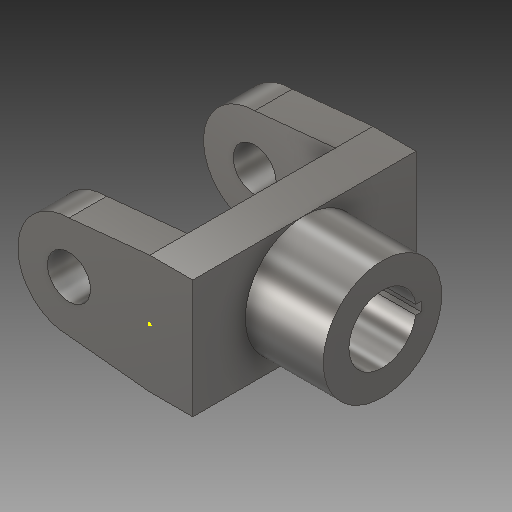
# Autodesk Inventor part: Fork 2 Off
Saved by Autodesk Inventor 2018 (Build 220112000, 112)
## iProperties
Created: 2018-09-13
Part Number: Fork 2 Off
Material: Stainless Steel
Document SubType Name: Modeling
Designer: Ajay Sharma
Density: 8 g/cm^3
Appearance: Semi-Polished
Author: Ajay Sharma
Autodesk Inventor part; units mm, degrees
ref_plane "YZ Plane" through (0, 0, 0) normal (1, 0, 0) x (0, 1, 0)
ref_plane "XZ Plane" through (0, 0, 0) normal (0, 1, 0) x (-1, 0, 0)
ref_plane "XY Plane" through (0, 0, 0) normal (0, 0, 1) x (1, 0, 0)
sketch "Sketch1" plane through (0, 0, 0) normal (1, 0, 0) x (0, 1, 0)
  line L0 (0, 116.2) -> (0, -116.2) projected
  line L1 (-61.6, 0) -> (61.6, 0) projected
  line L2 (44, 83) -> (-44, 83)
  line L3 (-44, 83) -> (-44, -83)
  line L4 (-44, -83) -> (44, -83)
  line L5 (44, -83) -> (44, 83)
  point P0 (0, 0)
  dimension "d0" = 166
  dimension "d1" = 88
  constraints: 8 end point, 2 parallel, 1 horizontal, 1 perpendicular, 2 other
  measures "d0" distance of L4.end L2.start
  measures "d1" distance of L2.start L2.end
extrude "Extrusion1" add sketch "Sketch1" along normal blind 32
sketch "Sketch2" plane through (32, 0, 0) normal (1, 0, 0) x (0, 0, -1)
  line L0 (-116.2, 0) -> (116.2, 0) projected
  line L1 (0, -61.6) -> (0, 61.6) projected
  circle A0 centre (0, 0) radius 44
  arc A1 (24.7538, 3.5) -> (24.7538, -3.5) centre (0, 0) ccw
  line L2 (25, 0) -> (29, 0)
  line L3 (29, 0) -> (29, 3.5)
  line L4 (29, 3.5) -> (24.7538, 3.5)
  arc A2 (24.7538, 3.5) -> (24.7538, -3.5) centre (0, 0) ccw
  line L5 (29, 0) -> (29, -3.5)
  line L6 (29, -3.5) -> (24.7538, -3.5)
  dimension "d4" = 88
  dimension "d5" = 50
  dimension "d6" = 4
  dimension "d7" = 3.5
  constraints: 10 end point, 4 point on circle, 3 centre point, 2 coincident, 2 perpendicular, 2 point on line, 2 symmetric about line, 1 other
  measures "d4" diameter of A0
  measures "d5" diameter of A1
  measures "d6" distance of L2.start L2.end
  measures "d7" distance of L2.end L3.end
extrude "Extrusion2" add sketch "Sketch2" along normal blind 58 contours L3 L4 A1 L1 A0 L0 | L0 A0 L1 A1 L6 L5 | A1 L1 A0 L0 | L0 A0 L1 A1
sketch "Sketch3" plane through (0, 0, 0) normal (-1, 0, 0) x (0, 0, 1)
  line L0 (-116.2, 0) -> (116.2, 0) projected
  line L1 (0, 61.6) -> (0, -61.6) projected
  line L2 (-83, 44) -> (83, 44) projected
  line L3 (83, -44) -> (-83, -44) projected
  line L4 (-83, 44) -> (-55, 44)
  line L5 (-55, 44) -> (-55, -44)
  line L6 (-55, -44) -> (-83, -44)
  line L7 (-83, -44) -> (-83, 44)
  line L8 (0, 44) -> (83, 44) projected
  line L9 (83, 44) -> (55, 44)
  line L10 (55, 44) -> (55, -44)
  line L11 (55, -44) -> (83, -44)
  line L12 (83, -44) -> (83, 44)
  point P0 (0, 0)
  dimension "d10" = 28
  dimension "d11" = 28
  constraints: 16 end point, 4 parallel, 2 horizontal, 2 perpendicular, 2 point on line
  measures "d10" distance from line of L5 L2.start
  measures "d11" distance from line of L10 L2.end
extrude "Extrusion3" add sketch "Sketch3" along normal blind 98 contours L7 L2 L5 L0 | L0 L5 L3 L7 | L10 L2 L12 L0 | L0 L12 L3 L10
sketch "Sketch4" plane through (32, -44, 83) normal (0, 0, 1) x (1, 0, 0)
  point P0 (-32, 44)
sketch "Sketch5" plane through (32, -44, 83) normal (0, 0, 1) x (1, 0, 0)
  circle A0 centre (-92, 44) radius 38
  line L0 (-92, 6) -> (-32, 0)
  line L1 (-130, 0) -> (0, 0) projected
  line L2 (-32, 88) -> (-32, 0) projected
  line L3 (-32, 88) -> (-92, 82)
  line L4 (0, 88) -> (-130, 88) projected
  line L5 (-32, 88) -> (-130, 88)
  line L6 (-130, 0) -> (-130, 88) projected
  line L7 (-130, 88) -> (-130, 0)
  line L8 (-130, 0) -> (-32, 0)
  point P0 (-32, 44)
  dimension "d14" = 76
  constraints: 10 end point, 2 collinear, 2 point on circle, 1 centre point, 1 perpendicular, 1 point on line
  measures "d14" diameter of A0
extrude "Extrusion4" cut sketch "Sketch5" against normal through all contours A0 L6 L4 L3 | L0 L1 L6 A0
sketch "Sketch6" plane through (32, -44, 83) normal (0, 0, 1) x (1, 0, 0)
  arc A0 (-92, 82) -> (-92, 6) centre (-92, 44) ccw projected
  circle A1 centre (-92, 44) radius 16
  point P0 (-32, 44)
  dimension "d17" = 32
  constraints: 1 centre point, 1 coincident
  measures "d17" diameter of A1
extrude "Extrusion5" cut sketch "Sketch6" against normal through all
body "Solid1"
